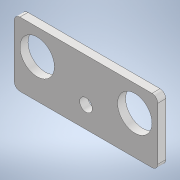
# Autodesk Inventor part: bok
Saved by Autodesk Inventor 2022.3 (Build 263350000, 350)
## iProperties
Created: 2022-12-14
Part Number: bok
Material: Generic
Document SubType Name: Modeling
Designer: komputer
Density: 1 g/cm^3
Appearance: Default
Author: komputer
Autodesk Inventor part; units mm, degrees
ref_plane "YZ Plane" through (0, 0, 0) normal (1, 0, 0) x (0, 1, 0)
ref_plane "XZ Plane" through (0, 0, 0) normal (0, 1, 0) x (-1, 0, 0)
ref_plane "XY Plane" through (0, 0, 0) normal (0, 0, 1) x (1, 0, 0)
sketch "Sketch1" plane through (0, 0, 0) normal (0, 0, 1) x (1, 0, 0)
  line L0 (-8.0811, -5.1131) -> (16.9189, -5.1131)
  line L1 (16.9189, -5.1131) -> (16.9189, 19.8869)
  line L2 (16.9189, 19.8869) -> (-8.0811, 19.8869)
  line L3 (-8.0811, 19.8869) -> (-8.0811, -5.1131)
  line L4 (-8.0811, -5.1131) -> (-7.0811, -5.1131)
  line L5 (-7.0811, -5.1131) -> (-7.0811, -4.1131)
  line L6 (-7.0811, -4.1131) -> (-8.0811, -4.1131)
  line L7 (-8.0811, -4.1131) -> (-8.0811, -5.1131)
  line L8 (16.9189, 19.8869) -> (15.9189, 19.8869)
  line L9 (15.9189, 19.8869) -> (15.9189, 18.8869)
  line L10 (15.9189, 18.8869) -> (16.9189, 18.8869)
  line L11 (16.9189, 18.8869) -> (16.9189, 19.8869)
  line L12 (-7.0811, -4.1131) -> (15.9189, -4.1131)
  line L13 (15.9189, -4.1131) -> (15.9189, 18.8869)
  line L14 (15.9189, 18.8869) -> (-7.0811, 18.8869)
  line L15 (-7.0811, 18.8869) -> (-7.0811, -4.1131)
  line L16 (-7.0811, -4.1131) -> (-1.0811, -4.1131)
  line L17 (-1.0811, -4.1131) -> (-1.0811, 17.1845)
  line L18 (-1.0811, 17.1845) -> (-7.0811, 17.1845)
  line L19 (-7.0811, 17.1845) -> (-7.0811, -4.1131)
  line L20 (15.9189, -4.1131) -> (9.9189, -4.1131)
  line L21 (9.9189, -4.1131) -> (9.9189, 17.1845)
  line L22 (9.9189, 17.1845) -> (15.9189, 17.1845)
  line L23 (15.9189, 17.1845) -> (15.9189, -4.1131)
  circle A0 centre (4.4189, 0.3869) radius 5.5
  line L24 (4.4189, 0.3869) -> (15.9189, 0.3869)
  line L25 (4.4189, 0.3869) -> (-8.0811, 0.3869)
  circle A1 centre (-4.0811, 3.3869) radius 3
  circle A2 centre (12.9189, 3.3869) radius 3
  circle A3 centre (4.4189, 0.3869) radius 5
  line L26 (4.4189, -4.6131) -> (4.4189, -3.3131)
  line L27 (4.4189, -3.3131) -> (16.9189, -3.3131)
  line L28 (4.4189, -3.3131) -> (-8.0811, -3.3131)
  line L29 (-4.0811, 6.3869) -> (-4.0811, 8.3869)
  line L30 (-4.0811, 8.3869) -> (16.9189, 8.3869)
  line L31 (-4.0811, 8.3869) -> (-8.0811, 8.3869)
  point P0 (0, 0)
  point P1 (0.3495, -3.3131)
  point P2 (8.4883, -3.3131)
  dimension "d8" = 10
  dimension "d0" = 25
  dimension "d1" = 25
  dimension "d2" = 1
  dimension "d3" = 1
  dimension "d4" = 1
  dimension "d5" = 1
  dimension "d6" = 6
  dimension "d7" = 6
  dimension "d9" = 1.3
  dimension "d10" = 2
  constraints: 64 end point, 12 parallel, 10 perpendicular, 9 point on line, 7 horizontal, 6 tangent, 3 vertical, 2 centre point, 2 vertical alignment, 1 coincident, 4 other
  measures "d0" distance of L2.end L1.end
  measures "d1" distance of L1.end L0.end
  measures "d2" distance of L6.end L5.end
  measures "d3" distance of L10.end L9.end
  measures "d4" distance of L9.end L8.end
  measures "d5" distance of L4.end L5.end
  measures "d6" distance of L18.end L17.end
  measures "d7" distance of L21.end L22.end
  measures "d9" distance of L26.start L26.end
  measures "d10" distance of L29.start L29.end
extrude "Extrusion1" add sketch "Sketch1" against normal blind 1 contours L3 L25 L15 L28 | L15 L25 L17 L28 | L3 L31 L15 L25 | L27 L13 L30 L1 | L28 L17 A0 | A0 L21 L27 | L15 A1 L25 | L27 L21 L24 L13 | L25 A1 L17 | L17 L30 L21 A0 | L21 A2 L24 | L15 L31 L29 A1 | L13 A2 L21 L30 | L24 A2 L13 | A1 L29 L30 L17
sketch "Sketch3" plane through (0, 0, 0) normal (0, 0, 1) x (1, 0, 0)
  line L0 (-8.0811, 8.3869) -> (-8.0811, -3.3131) projected
  line L1 (-8.0811, -3.3131) -> (0.3495, -3.3131) projected
  arc A0 (8.4883, -3.3131) -> (0.3495, -3.3131) centre (4.4189, 0.3869) ccw projected
  line L2 (8.4883, -3.3131) -> (16.9189, -3.3131) projected
  line L3 (16.9189, -3.3131) -> (16.9189, 8.3869) projected
  line L4 (16.9189, 8.3869) -> (-8.0811, 8.3869) projected
  circle A1 centre (12.9189, 3.3869) radius 3 projected
  circle A2 centre (-4.0811, 3.3869) radius 3 projected
  circle A3 centre (4.4189, 0.3869) radius 1.1 projected
  arc A4 (8.4883, -3.3131) -> (0.3495, -3.3131) centre (4.4189, 0.3869) ccw projected
  line L5 (16.9189, -3.3131) -> (8.4883, -3.3131) projected
  line L6 (0.3495, -3.3131) -> (8.4883, -3.3131)
  point P0 (0, 0)
  constraints: 2 end point, 1 horizontal
extrude "Extrusion2" add sketch "Sketch3" against normal blind 1 contours A0 L6
sketch "Sketch4" plane through (0, 0, -1) normal (0, 0, -1) x (-1, 0, 0)
  circle A0 centre (-4.4189, 0.3869) radius 1.1 projected
  line L0 (8.0811, -3.3131) -> (8.0811, 8.3869) projected
  line L1 (8.0811, 8.3869) -> (-16.9189, 8.3869) projected
  line L2 (-16.9189, 8.3869) -> (-16.9189, -3.3131) projected
  line L3 (-16.9189, -3.3131) -> (8.0811, -3.3131) projected
  circle A1 centre (-12.9189, 3.3869) radius 3 projected
  circle A2 centre (4.0811, 3.3869) radius 3 projected
  circle A3 centre (-12.9189, 3.3869) radius 4
  line L4 (-16.9189, 8.3869) -> (-16.9189, -3.3131) projected
  line L5 (-12.9189, 7.3869) -> (-12.9189, 8.3869)
  line L6 (-12.9189, 7.8869) -> (-16.9189, 7.8869)
  line L7 (-12.9189, 7.8869) -> (8.0811, 7.8869)
  line L8 (8.0811, -3.3131) -> (8.0811, 8.3869) projected
  point P0 (0, 0)
  point P1 (8.0811, 7.8869)
  constraints: 6 end point, 4 point on line, 1 coincident, 1 midpoint, 1 parallel, 1 perpendicular, 1 vertical, 1 vertical alignment, 2 other
extrude "Extrusion3" cut sketch "Sketch4" against normal blind 1 contours L7 L5 L1 L0 | L6 L2 L1 L5
fillet "Fillet1" radius 1 4 edges at (16.9189, 7.8869, -0.5) (16.9189, -3.3131, -0.5) (-8.0811, 7.8869, -0.5) (-8.0811, -3.3131, -0.5)
sketch "Sketch5" plane through (0, 0, -1) normal (0, 0, -1) x (-1, 0, 0)
  circle A0 centre (4.0811, 3.3869) radius 3 projected
  circle A1 centre (-12.9189, 3.3869) radius 3 projected
  circle A2 centre (-4.4189, 0.3869) radius 1.1 projected
  arc A3 (7.0811, -3.3131) -> (8.0811, -2.3131) centre (7.0811, -2.3131) ccw projected
  line L0 (8.0811, -2.3131) -> (8.0811, 6.8869) projected
  arc A4 (8.0811, 6.8869) -> (7.0811, 7.8869) centre (7.0811, 6.8869) ccw projected
  line L1 (7.0811, 7.8869) -> (-15.9189, 7.8869) projected
  arc A5 (-15.9189, 7.8869) -> (-16.9189, 6.8869) centre (-15.9189, 6.8869) ccw projected
  line L2 (-16.9189, 6.8869) -> (-16.9189, -2.3131) projected
  arc A6 (-16.9189, -2.3131) -> (-15.9189, -3.3131) centre (-15.9189, -2.3131) ccw projected
  line L3 (-15.9189, -3.3131) -> (7.0811, -3.3131) projected
  point P0 (0, 0)
extrude "Extrusion4" add sketch "Sketch5" along normal blind 0.2
sketch "Sketch6" plane through (0, 0, 0) normal (0, 0, 1) x (1, 0, 0)
  arc A0 (-8.0811, -2.3131) -> (-7.0811, -3.3131) centre (-7.0811, -2.3131) ccw projected
  line L0 (-7.0811, -3.3131) -> (15.9189, -3.3131) projected
  arc A1 (15.9189, -3.3131) -> (16.9189, -2.3131) centre (15.9189, -2.3131) ccw projected
  line L1 (16.9189, -2.3131) -> (16.9189, 6.8869) projected
  arc A2 (16.9189, 6.8869) -> (15.9189, 7.8869) centre (15.9189, 6.8869) ccw projected
  line L2 (15.9189, 7.8869) -> (-7.0811, 7.8869) projected
  arc A3 (-7.0811, 7.8869) -> (-8.0811, 6.8869) centre (-7.0811, 6.8869) ccw projected
  line L3 (-8.0811, 6.8869) -> (-8.0811, -2.3131) projected
  circle A4 centre (4.4189, 0.3869) radius 1.1 projected
  circle A5 centre (12.9189, 3.3869) radius 3 projected
  circle A6 centre (-4.0811, 3.3869) radius 3 projected
  point P0 (0, 0)
extrude "Extrusion5" add sketch "Sketch6" along normal blind 0.2
body "Solid1"
